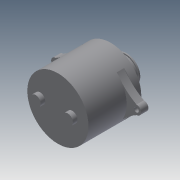
# Autodesk Inventor part: alternator
Saved by Autodesk Inventor 2015 (Build 190159000, 159)
## iProperties
Created: 2014-08-31
Part Number: alternator
Material: Generic
Document SubType Name: Modeling
Designer: shohei
Density: 1 g/cm^3
Appearance: Default
Author: shohei
Autodesk Inventor part; units mm, degrees
ref_plane "YZ Plane" through (0, 0, 0) normal (1, 0, 0) x (0, 1, 0)
ref_plane "XZ Plane" through (0, 0, 0) normal (0, 1, 0) x (-1, 0, 0)
ref_plane "XY Plane" through (0, 0, 0) normal (0, 0, 1) x (1, 0, 0)
sketch "Sketch1" plane through (0, 0, 0) normal (0, 1, 0) x (-1, 0, 0)
  circle A0 centre (0, 0) radius 67.183
  dimension "d0" = 134.366
  constraints: 1 centre point, 1 coincident
  measures "d0" diameter of A0
extrude "Extrusion1" add sketch "Sketch1" along normal blind 83.82
sketch "Sketch2" plane through (0, 83.82, 0) normal (0, 1, 0) x (1, 0, 0)
  arc A0 (-88.791, 10) -> (-88.791, -10) centre (-88.773, 0) ccw
  line L0 (0, 169.5617) -> (0, -169.5617) projected
  arc A1 (88.791, -10) -> (88.791, 10) centre (88.773, 0) ccw
  arc A2 (-45.3457, -49.5714) -> (-88.791, -10) centre (-150.2545, -121.1155) ccw
  line L1 (-210.3564, 0) -> (210.3564, 0) projected
  arc A3 (-88.791, 10) -> (-45.3457, 49.5714) centre (-150.2545, 121.1155) ccw
  arc A4 (88.791, -10) -> (45.3457, -49.5714) centre (150.2545, -121.1155) ccw
  arc A5 (45.3457, 49.5714) -> (88.791, 10) centre (150.2545, 121.1155) ccw
  circle A6 centre (88.773, 0) radius 5
  circle A7 centre (-88.773, 0) radius 5
  arc A8 (-45.3457, -49.5714) -> (45.3457, -49.5714) centre (0, 0) ccw
  arc A9 (45.3457, 49.5714) -> (-45.3457, 49.5714) centre (0, 0) ccw
  dimension "d4" = 88.773
  dimension "d5" = 20
  dimension "d6" = 10
  dimension "d7" = 10
  constraints: 16 point on circle, 10 centre point, 10 symmetric about line, 3 coincident, 1 point on line, 4 other
  measures "d4" distance of A8.centre A0.centre
  measures "d5" diameter of A0
  measures "d6" diameter of A6
  measures "d7" diameter of A7
extrude "Extrusion2" add sketch "Sketch2" along normal blind 16.256 contours A3 A9 L0 L1 A7 A0 | L1 A7 L0 A8 A2 A0 | A9 A5 A1 L1 A6 L0 | L1 A6 A1 A4 A8 L0
sketch "Sketch3" plane through (0, 0, 0) normal (0, -1, 0) x (1, 0, 0)
  circle A0 centre (0, 0) radius 67.183 projected
  circle A1 centre (-39.2802, 0) radius 11.4333
  circle A2 centre (31.4242, 0) radius 11.6008
  line L0 (-138.2822, 0) -> (138.2822, 0) projected
  line L1 (0, -94.0562) -> (0, 94.0562) projected
  constraints: 2 centre point
extrude "Extrusion3" add sketch "Sketch3" along normal blind 10 contours L0 A2 | A2 L0 | L0 A1 | A1 L0
sketch "Sketch4" plane through (0, 100.076, 0) normal (0, 1, 0) x (1, 0, 0)
  circle A0 centre (0, 0) radius 67.183
  dimension "d12" = 134.366
  constraints: 1 centre point, 1 coincident
  measures "d12" diameter of A0
extrude "Extrusion4" add sketch "Sketch4" along normal blind 15.875
sketch "Sketch5" plane through (0, 115.951, 0) normal (0, 1, 0) x (1, 0, 0)
  circle A0 centre (0, 0) radius 30
  dimension "d17" = 60
  constraints: 1 centre point, 1 coincident
  measures "d17" diameter of A0
extrude "Extrusion5" add sketch "Sketch5" along normal blind 2.921
sketch "Sketch6" plane through (0, 118.872, 0) normal (0, 1, 0) x (1, 0, 0)
  circle A0 centre (0, 0) radius 27.5
  dimension "d18" = 55
  constraints: 1 centre point, 1 coincident
  measures "d18" diameter of A0
extrude "Extrusion6" add sketch "Sketch6" along normal blind 29.21
sketch "Sketch7" plane through (0, 148.082, 0) normal (0, 1, 0) x (1, 0, 0)
  circle A0 centre (0, 0) radius 30
  dimension "d21" = 60
  constraints: 1 centre point, 1 coincident
  measures "d21" diameter of A0
extrude "Extrusion7" add sketch "Sketch7" along normal blind 2.921
body "Solid1"
